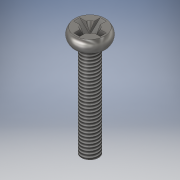
# Autodesk Inventor part: M3x16
Saved by Autodesk Inventor 2019 (Build 230136000, 136)
## iProperties
Created: 2021-01-02
Part Number: M3x16
Material: Сталь, литейная
Document SubType Name: Modeling
Designer: Professional
Density: 7.85 g/cm^3
Appearance: С умеренной полировкой
Author: Professional
Autodesk Inventor part; units mm, degrees
ref_plane "YZ Plane" through (0, 0, 0) normal (1, 0, 0) x (0, 1, 0)
ref_plane "XZ Plane" through (0, 0, 0) normal (0, 1, 0) x (-1, 0, 0)
ref_plane "XY Plane" through (0, 0, 0) normal (0, 0, 1) x (1, 0, 0)
sketch "Эскиз3" plane through (0, 0, 0) normal (0, 0, 1) x (1, 0, 0)
  line L0 (-1.4, 0) -> (-1.4, -16)
  line L1 (-1.4, -16) -> (0, -16)
  line L2 (0, -16) -> (0, 2)
  line L3 (-1.4, 0) -> (-2.5, 0)
  arc A0 (-2.5, 2) -> (-2.5, 0) centre (-1.4, 1) ccw
  line L4 (-1.3, 2) -> (-0.5, 0.4)
  line L5 (-0.5, 0.4) -> (0, 0.4)
  line L6 (-2.5, 2) -> (-1.3, 2)
  point P0 (0, 0)
  dimension "d4" = 2.8
  dimension "d6" = 1
  dimension "d7" = 5
  dimension "d8" = 16
  dimension "d10" = 2
  dimension "d12" = 2.6
  dimension "d13" = 0.4
  dimension "d14" = 1
  constraints: 14 end point, 2 horizontal, 2 horizontal alignment, 2 perpendicular, 2 point on circle, 2 point on line, 2 vertical, 1 centre point, 1 vertical alignment
  measures "d4" diameter of L0 L2
  measures "d6" distance of L0.start A0.centre
  measures "d7" diameter of L6.start L2
  measures "d8" distance between parallel lines of L1 L3
  measures "d10" distance of L3.end L6.start
  measures "d12" diameter of L4.start L2
  measures "d13" distance from line of L5 L0.start
  measures "d14" diameter of L4.end L2
revolve "Вращение1" add sketch "Эскиз3" angle 360 about axis through (0, -16, 0) along (0, 1, 0)
sketch "Эскиз5" plane through (0, 0, 0) normal (0, 0, 1) x (1, 0, 0)
  line L0 (0.5, 0.4) -> (-0.5, 0.4) projected
  line L1 (-0.5, 0.4) -> (-2.2, 2)
  line L2 (2.5, 2) -> (-2.5, 2) projected
  line L3 (-2.2, 2) -> (0, 2)
  line L4 (1.3, 2) -> (-1.3, 2) projected
  line L5 (0, 0.4) -> (-0.5, 0.4)
  line L6 (0, 0.4) -> (0, 2)
  point P0 (0, 0)
  dimension "d15" = 2.2
  constraints: 8 end point, 1 midpoint, 1 parallel, 1 perpendicular, 1 point on line
  measures "d15" distance of L3.end L1.end
extrude "Выдавливание2" cut sketch "Эскиз5" along normal mid plane 1
pattern_circular "Круговой массив1" count 4 over 360 about axis through (0, -10, 0) along (0, 1, 0) of "Выдавливание2"
thread "Резьба1" size "M3x0.5" class "6g" standard "ANSI Metric M Profile" full length
